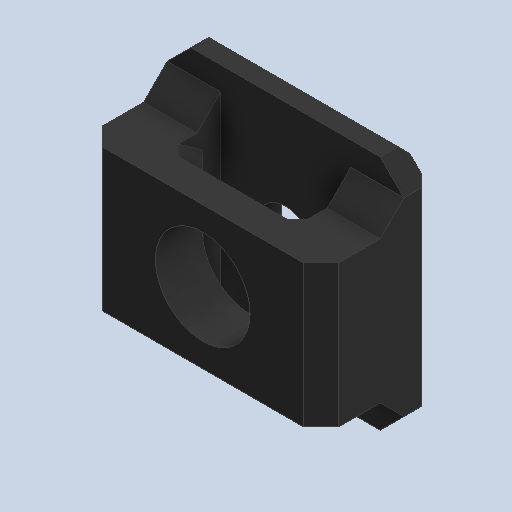
# Autodesk Inventor part: CableHolder
Saved by Autodesk Inventor 2022 (Build 260153000, 153)
## iProperties
Created: 2020-07-16
Part Number: CableHolder
Material: Generic
Document SubType Name: Modeling
Designer: CASE-SMALL2
Density: 1 g/cm^3
Appearance: Default
Author: CASE-SMALL2
## iProperties of the stored document _3DPrint.ipt
Created: 2021-02-25
Part Number: _3DPrint
Material: Generic
Document SubType Name: Modeling
Designer: Viktor
Density: 1 g/cm^3
Appearance: Default
Author: Viktor
Autodesk Inventor part; units mm, degrees
ref_plane "YZ Plane" through (0, 0, 0) normal (1, 0, 0) x (0, 1, 0)
ref_plane "XZ Plane" through (0, 0, 0) normal (0, 1, 0) x (-1, 0, 0)
ref_plane "XY Plane" through (0, 0, 0) normal (0, 0, 1) x (1, 0, 0)
sketch "Sketch1" plane through (0, 0, 0) normal (0, 0, 1) x (1, 0, 0)
  line L0 (-10, -10) -> (10, -10)
  line L1 (10, -10) -> (10, 10)
  line L2 (10, 10) -> (-10, 10)
  line L3 (-10, 10) -> (-10, -10)
  line L4 (-10, -10) -> (10, 10) construction
  line L5 (10, -10) -> (-10, 10) construction
  circle A0 centre (0, 0) radius 2.4
  dimension "d0" = 20
  dimension "d1" = 20
  dimension "d2" = 4.8
  constraints: 12 end point, 2 midpoint, 2 parallel, 1 centre point, 1 coincident, 1 horizontal, 1 perpendicular
  measures "d0" distance between parallel lines of L0 L2
  measures "d1" distance between parallel lines of L1 L3
  measures "d2" diameter of A0
extrude "Extrusion1" add sketch "Sketch1" along normal blind 2
chamfer "Chamfer1" distance 0.5 angle 45 4 edges at (10, 0, 0) (0, 10, 0) (-10, 0, 0) (0, -10, 0)
sketch "Sketch2" plane through (0, 0, 2) normal (0, 0, 1) x (1, 0, 0)
  line L0 (10, 10) -> (10, -10) projected
  line L1 (-10, -6) -> (10, -6)
  line L2 (10, -6) -> (10, 6)
  line L3 (10, 6) -> (-10, 6)
  line L4 (-10, 6) -> (-10, -6)
  line L5 (-10, -6) -> (10, 6) construction
  line L6 (10, -6) -> (-10, 6) construction
  point P0 (0, 0)
  point P1 (10, -6)
  dimension "d8" = 12
  constraints: 12 end point, 2 midpoint, 2 parallel, 1 horizontal, 1 perpendicular, 1 point on line
  measures "d8" distance between parallel lines of L1 L3
extrude "Extrusion2" add sketch "Sketch2" along normal blind 7
sketch "Sketch5" plane through (-10, -6, 2) normal (0, -1, 0) x (1, 0, 0)
  line L0 (20, 0) -> (0, 0) projected
  line L1 (4.5, 0) -> (15.5, 0)
  line L2 (15.5, 0) -> (15.5, 3)
  line L3 (15.5, 3) -> (4.5, 3)
  line L4 (4.5, 3) -> (4.5, 0)
  line L5 (0, 0) -> (0, 7) projected
  line L6 (20, 0) -> (20, 7) projected
  point P0 (10, -2)
  dimension "d18" = 3
  dimension "d19" = 4.5
  dimension "d20" = 4.5
  constraints: 8 end point, 2 parallel, 1 horizontal, 1 perpendicular, 1 point on line
  measures "d18" distance between parallel lines of L0 L3
  measures "d19" distance between parallel lines of L5 L4
  measures "d20" distance between parallel lines of L6 L2
extrude "Extrusion4" cut sketch "Sketch5" against normal through all
sketch "Sketch6" plane through (0, 0, 9) normal (0, 0, 1) x (1, 0, 0)
  circle A0 centre (0, 0) radius 2.4 construction
  circle A1 centre (0, 0) radius 4
  dimension "d23" = 8
  constraints: 1 centre point, 1 coincident
  measures "d23" diameter of A1
extrude "Extrusion5" cut sketch "Sketch6" against normal up to surface (7 mm away)
chamfer "Chamfer4" distance 1.5 angle 45 2 edges at (-5.5, 0, 5) (5.5, 0, 5)
chamfer "Chamfer5" distance 1.5 angle 45 6 edges at (0, -6, 5) (0, 6, 5) (-4.75, -6, 4.25) (4.75, -6, 4.2501) (4.75, 6, 4.25) (-4.75, 6, 4.2501)
chamfer "Chamfer6" distance 1.5 angle 45 2 edges at (-10, 0, 9) (10, 0, 9)
chamfer "Chamfer7" distance 2 angle 45 8 edges at (10, 10, 1.25) (-10, 10, 1.25) (-10, -10, 1.25) (10, -10, 1.25) (7.75, -6, 2) (-7.75, -6, 2) (-7.75, 6, 2) (7.75, 6, 2)
equation "\"d20\" = d19"
body "Solid1"
